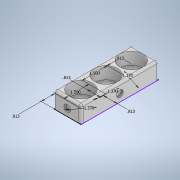
# Autodesk Inventor part: paint_holder_w_magnet
Saved by Autodesk Inventor 2021 (Build 250183000, 183)
## iProperties
Created: 2020-12-04
Part Number: paint_holder_w_magnet
Material: Generic
Document SubType Name: Modeling
Designer: Patrick
Density: 1 g/cm^3
Appearance: Default
Author: Patrick
## iProperties of the stored document _3DPrint.ipt
Created: 2020-12-04
Part Number: _3DPrint
Material: Generic
Document SubType Name: Modeling
Designer: Patrick
Density: 1 g/cm^3
Appearance: Default
Author: Patrick
Autodesk Inventor part; units mm, degrees
ref_plane "YZ Plane" through (0, 0, 0) normal (1, 0, 0) x (0, 1, 0)
ref_plane "XZ Plane" through (0, 0, 0) normal (0, 1, 0) x (-1, 0, 0)
ref_plane "XY Plane" through (0, 0, 0) normal (0, 0, 1) x (1, 0, 0)
sketch "Sketch1" plane through (0, 0, 0) normal (0, 1, 0) x (-1, 0, 0)
  circle A0 centre (0, 0) radius 17.399
  circle A1 centre (0, -38.1) radius 17.399
  circle A2 centre (0, -76.2) radius 17.399
  line L0 (20.65, 20.65) -> (-20.65, 20.65)
  line L1 (-20.65, 20.65) -> (-20.65, -96.85)
  line L2 (-20.65, -96.85) -> (20.65, -96.85)
  line L3 (20.65, -96.85) -> (20.65, 20.65)
  dimension "d0" = 34.798
  dimension "d1" = 34.798
  dimension "d2" = 38.1
  dimension "d3" = 34.798
  dimension "d4" = 38.1
  dimension "d5" = 20.65
  dimension "d6" = 20.65
  dimension "d7" = 20.65
  dimension "d8" = 20.65
  constraints: 8 end point, 3 centre point, 2 parallel, 1 coincident, 1 horizontal, 1 perpendicular
  measures "d0" diameter of A0
  measures "d1" diameter of A1
  measures "d2" distance of A1.centre point (0, 0)
  measures "d3" diameter of A2
  measures "d4" distance of A2.centre A1.centre
  measures "d5" distance from line of L0 point (0, 0)
  measures "d6" distance from line of L2 A2.centre
  measures "d7" distance from line of L1 A1.centre
  measures "d8" distance from line of L3 A1.centre
extrude "Extrusion1" add sketch "Sketch1" along normal blind 25
extrude "Extrusion2" add sketch "Sketch1" along normal blind 6.35 contours A0 | A1 | A2
fillet "Fillet1" radius 3.175 8 edges at (20.65, 12.5, 20.65) (-20.65, 12.5, 20.65) (20.65, 12.5, -96.85) (-20.65, 12.5, -96.85) (0, 25, -96.85) (0, 25, 20.65) (20.65, 25, -38.1) (-20.65, 25, -38.1)
sketch "Sketch3" plane through (-20.65, 0, -93.675) normal (-1, 0, 0) x (0, 0, 1)
  circle A0 centre (55.5752, 10.9157) radius 5
  line L0 (0, 0) -> (0, 21.825) projected
  line L1 (0, 21.825) -> (111.15, 21.825) projected
  point P0 (93.675, 0)
  dimension "d19" = 10
  dimension "d20" = 55.5752
  dimension "d21" = 10.9093
  constraints: 1 centre point
  measures "d19" diameter of A0
  measures "d20" distance from line of L0 A0.centre
  measures "d21" distance from line of L1 A0.centre
extrude "Extrusion4" cut sketch "Sketch3" against normal blind 3
sketch "Sketch4" plane through (-17.475, 0, 20.65) normal (0, 0, 1) x (1, 0, 0)
  circle A0 centre (17.4752, 10.9157) radius 5
  line L0 (0, 0) -> (0, 21.825) projected
  line L1 (0, 21.825) -> (34.95, 21.825) projected
  point P0 (17.475, 0)
  dimension "d24" = 10
  dimension "d25" = 17.4752
  dimension "d26" = 10.9093
  constraints: 1 centre point
  measures "d24" diameter of A0
  measures "d25" distance from line of L0 A0.centre
  measures "d26" distance from line of L1 A0.centre
extrude "Extrusion5" cut sketch "Sketch4" against normal blind 3
sketch "Sketch5" plane through (20.65, 0, 17.475) normal (1, 0, 0) x (0, 0, -1)
  circle A0 centre (55.5748, 10.9157) radius 5 projected
  circle A1 centre (55.5748, 10.9157) radius 5
  point P0 (17.475, 0)
  dimension "d29" = 10
  constraints: 1 centre point, 1 coincident
  measures "d29" diameter of A1
extrude "Extrusion6" cut sketch "Sketch5" against normal blind 3
sketch "Sketch6" plane through (17.475, 0, -96.85) normal (0, 0, -1) x (-1, 0, 0)
  circle A0 centre (17.4748, 10.9157) radius 5 projected
  circle A1 centre (17.4748, 10.9157) radius 5
  point P0 (17.475, 0)
  constraints: 1 centre point, 1 coincident
extrude "Extrusion7" cut sketch "Sketch6" against normal blind 3
body "Solid1"
